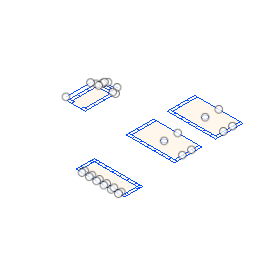
Plano_caja v3 (Autodesk Fusion 360 design; units mm, degrees)
Autodesk Fusion 360 part; units mm, degrees
sketch "Cara_base" plane through (0, 0, 0) normal (0, 1, 0) x (1, 0, 0)
  line L0 (25, -25) -> (78, -25)
  line L1 (78, -25) -> (78, -45)
  line L2 (78, -45) -> (25, -45)
  line L3 (25, -45) -> (25, -25)
  line L4 (25, -45) -> (28, -45)
  line L5 (28, -25) -> (28, -45)
  line L6 (78, -45) -> (75, -45)
  line L7 (75, -25) -> (75, -45)
  line L8 (25, -25) -> (25, -28)
  line L9 (78, -28) -> (25, -28)
  line L10 (25, -45) -> (25, -42)
  line L11 (25, -42) -> (78, -42)
  line L12 (25, -25) -> (25, -30)
  line L13 (25, -30) -> (28, -30)
  line L14 (28, -40) -> (25, -40)
  line L15 (75, -30) -> (78, -30)
  line L16 (75, -40) -> (78, -40)
  line L17 (28, -25) -> (31.5, -25)
  line L18 (31.5, -25) -> (31.5, -28)
  line L19 (75, -28) -> (71.5, -28)
  line L20 (31.5, -28) -> (39.5, -28)
  line L21 (39.4691, -25) -> (39.5, -28)
  line L22 (39.5, -28) -> (47.5, -28)
  line L23 (47.5, -25) -> (47.5, -28)
  line L24 (47.5, -28) -> (55.5, -28)
  line L25 (55.5, -25) -> (55.5, -28)
  line L26 (55.5, -28) -> (63.5, -28)
  line L27 (63.5, -28) -> (63.5, -25)
  line L28 (63.5, -28) -> (71.5, -28)
  line L29 (71.5, -25) -> (71.5, -28)
  line L30 (31.5, -42) -> (31.5, -45)
  line L31 (39.4691, -42) -> (39.5, -45)
  line L32 (47.5, -42) -> (47.5, -45)
  line L33 (55.5, -42) -> (55.5, -45)
  line L34 (63.5, -45) -> (63.5, -42)
  line L35 (71.5, -42) -> (71.5, -45)
  dimension "d1" = 53
  dimension "d2" = 20
  dimension "d3" = 3.5
  dimension "d4" = 3.5
  dimension "d5" = 8
  dimension "d6" = 8
  dimension "d7" = 8
  dimension "d8" = 8
  dimension "d11" = 0
  dimension "d12" = -17
  constraint horizontal L0
  constraint vertical L1
  constraint horizontal L2
  constraint vertical L3
  constraint coincident L2 L4.end
  constraint coincident L0 L5.start
  constraint perpendicular L0 L5
  constraint coincident L2 L6.end
  constraint coincident L0 L7.start
  constraint perpendicular L2 L7
  constraint coincident L3 L8.end
  constraint coincident L1 L9.start
  constraint perpendicular L3 L9
  constraint coincident L3 L10.end
  constraint coincident L1 L11.end
  constraint perpendicular L1 L11
  constraint coincident L3 L12.end
  constraint coincident L5 L13.end
  constraint perpendicular L5 L13
  constraint coincident L3 L14.end
  constraint coincident L5 L14.start
  constraint perpendicular L3 L14
  constraint coincident L7 L15.start
  constraint coincident L1 L15.end
  constraint perpendicular L1 L15
  constraint coincident L7 L16.start
  constraint coincident L1 L16.end
  constraint perpendicular L1 L16
  constraint coincident L0 L17.end
  constraint coincident L9 L18.end
  constraint perpendicular L9 L18
  constraint coincident L7 L19.start
  constraint coincident L9 L19.start
  constraint perpendicular L7 L19
  constraint coincident L9 L20.end
  constraint coincident L0 L21.start
  constraint coincident L9 L22.end
  constraint coincident L0 L23.start
  constraint perpendicular L0 L23
  constraint coincident L9 L24.end
  constraint coincident L0 L25.start
  constraint perpendicular L0 L25
  constraint coincident L9 L26.end
  constraint coincident L0 L27.end
  constraint perpendicular L0 L27
  constraint coincident L0 L29.start
  constraint perpendicular L19 L29
  measures "d1" distance of L0.start L0.end
  measures "d2" distance of L0.start L2.end
  measures "d3" distance of L5.start L17.end
  measures "d4" distance of L19.start L19.end
  measures "d5" distance of L18.end L20.end L0.end
  measures "d6" distance of L20.end L22.end L0.end
  measures "d7" distance of L22.end L24.end L0.end
  measures "d8" distance of L24.end L26.end L0.end
extrude "Extrude1" add sketch "Cara_base" along normal blind 3 contours L0 L3 L5 L8 L9 L12 | L0 L5 L9 L17 L18 | L3 L5 L9 L12 L13 | L5 L7 L9 L11 L19 L20 L22 L24 L26 L28 | L0 L9 L21 L22 L23 | L3 L5 L11 L14 | L2 L3 L4 L5 L10 L11 | L0 L9 L25 L26 L27 | L2 L5 L11 L30 | L0 L7 L9 L19 L29 | L2 L11 L31 L32 | L0 L1 L7 L9 | L1 L7 L9 L15 | L2 L11 L33 L34 | L1 L7 L11 L16 | L2 L7 L11 L35 | L1 L2 L6 L7 L11 makes body 1
sketch "Cara_frontal" plane through (0, 0, 0) normal (0, 1, 0) x (1, 0, 0)
  line L0 (20, 15) -> (73, 15)
  line L1 (73, 15) -> (73, 45)
  line L2 (73, 45) -> (20, 45)
  line L3 (20, 45) -> (20, 15)
  line L4 (20, 15) -> (20, 18)
  line L5 (20, 18) -> (73, 18)
  line L6 (20, 18) -> (26.5, 18)
  line L7 (26.5, 18) -> (26.5, 15)
  line L8 (26.5, 15) -> (34.5, 15)
  line L9 (34.5, 15) -> (34.5, 18)
  line L10 (34.5, 15) -> (42.5, 15)
  line L11 (42.5, 15) -> (50.5, 15)
  line L12 (50.5, 15) -> (58.5, 15)
  line L13 (58.5, 15) -> (66.5, 15)
  line L14 (66.5, 15) -> (73, 15)
  line L15 (42.5, 18) -> (42.5, 15)
  line L16 (50.5, 18) -> (50.5, 15)
  line L17 (58.5, 18) -> (58.5, 15)
  line L18 (66.5, 18) -> (66.5, 15)
  line L19 (20, 45) -> (23, 45)
  line L20 (23, 45) -> (23, 36.5)
  line L21 (23, 36.5) -> (20, 36.5)
  line L22 (23, 36.5) -> (23, 26.5)
  line L23 (23, 26.5) -> (20, 26.5)
  line L24 (23, 26.5) -> (23, 18)
  line L25 (73, 26.5) -> (70, 26.5)
  line L26 (73, 36.5) -> (70, 36.5)
  line L27 (70, 45) -> (70, 18)
  line L28 (23, 45) -> (46.5, 45)
  circle A0 centre (46.5, 30) radius 2.5
  line L29 (26.5, 63) -> (26.5, 60)
  line L30 (73, 90) -> (20, 90)
  circle A1 centre (46.5, 75) radius 2.5
  line L31 (20, 90) -> (23, 90)
  line L32 (73, 60) -> (73, 90)
  line L33 (73, 71.5) -> (70, 71.5)
  line L34 (20, 63) -> (26.5, 63)
  line L35 (23, 81.5) -> (20, 81.5)
  line L36 (66.5, 60) -> (73, 60)
  line L37 (58.5, 60) -> (66.5, 60)
  line L38 (50.5, 60) -> (58.5, 60)
  line L39 (20, 60) -> (73, 60)
  line L40 (23, 81.5) -> (23, 71.5)
  line L41 (42.5, 60) -> (50.5, 60)
  line L42 (50.5, 63) -> (50.5, 60)
  line L43 (73, 81.5) -> (70, 81.5)
  line L44 (23, 71.5) -> (20, 71.5)
  line L45 (70, 90) -> (70, 63)
  line L46 (42.5, 63) -> (42.5, 60)
  line L47 (26.5, 60) -> (34.5, 60)
  line L48 (34.5, 60) -> (42.5, 60)
  line L49 (23, 71.5) -> (23, 63)
  line L50 (34.5, 60) -> (34.5, 63)
  line L51 (20, 60) -> (20, 63)
  line L52 (58.5, 63) -> (58.5, 60)
  line L53 (20, 90) -> (20, 60)
  line L54 (66.5, 63) -> (66.5, 60)
  line L55 (23, 90) -> (46.5, 90)
  line L56 (20, 63) -> (73, 63)
  line L57 (23, 90) -> (23, 81.5)
  dimension "d15" = 30
  dimension "d16" = 53
  dimension "d48" = 5
  dimension "d49" = 30
  dimension "d50" = 53
  dimension "d51" = 5
  constraint horizontal L0
  constraint vertical L1
  constraint horizontal L2
  constraint vertical L3
  constraint coincident L3 L4.end
  constraint coincident L1 L5.end
  constraint perpendicular L1 L5
  constraint coincident L5 L6.end
  constraint coincident L0 L7.end
  constraint perpendicular L0 L7
  constraint coincident L0 L8.end
  constraint coincident L5 L9.end
  constraint perpendicular L5 L9
  constraint coincident L0 L10.end
  constraint coincident L0 L11.end
  constraint coincident L0 L12.end
  constraint coincident L0 L13.end
  constraint coincident L5 L15.start
  constraint coincident L5 L16.start
  constraint coincident L5 L17.start
  constraint coincident L5 L18.start
  constraint coincident L2 L19.end
  constraint perpendicular L2 L20
  constraint coincident L3 L21.end
  constraint perpendicular L3 L21
  constraint perpendicular L21 L22
  constraint coincident L3 L23.end
  constraint perpendicular L3 L23
  constraint coincident L5 L24.end
  constraint coincident L1 L25.start
  constraint perpendicular L1 L25
  constraint coincident L1 L26.start
  constraint perpendicular L1 L26
  constraint coincident L2 L27.start
  constraint coincident L5 L27.end
  constraint perpendicular L5 L27
  constraint perpendicular L27 L28
  constraint horizontal L39
  constraint vertical L32
  constraint horizontal L30
  constraint vertical L53
  constraint coincident L34.start L53
  constraint coincident L56.end L32
  constraint perpendicular L32 L56
  constraint coincident L29.start L56
  constraint coincident L29.end L39
  constraint perpendicular L29 L39
  constraint coincident L47.end L39
  constraint coincident L50.end L56
  constraint perpendicular L50 L56
  constraint coincident L41.start L39
  constraint coincident L38.start L39
  constraint coincident L37.start L39
  constraint coincident L36.start L39
  constraint coincident L46.start L56
  constraint coincident L42.start L56
  constraint coincident L52.start L56
  constraint coincident L54.start L56
  constraint coincident L31.end L30
  constraint perpendicular L30 L57
  constraint coincident L35.end L53
  constraint perpendicular L35 L53
  constraint perpendicular L35 L40
  constraint coincident L44.end L53
  constraint perpendicular L44 L53
  constraint coincident L49.end L56
  constraint coincident L33.start L32
  constraint perpendicular L32 L33
  constraint coincident L43.start L32
  constraint perpendicular L32 L43
  constraint coincident L45.start L30
  constraint coincident L45.end L56
  constraint perpendicular L45 L56
  constraint perpendicular L45 L55
  measures "d15" distance of L0.start L2.end
  measures "d16" distance of L0.start L0.end
  measures "d48" diameter of A0
  measures "d49" distance of L39.start L30.end
  measures "d50" distance of L39.start L32.start
  measures "d51" diameter of A1
extrude "Extrude3" add sketch "Cara_frontal" along normal blind 3 separate body contours L0 L5 L7 L8 L9 | L2 L5 L6 L20 L22 L24 L27 L28 | L3 L21 L22 L23 | L0 L5 L11 L15 L16 | L0 L5 L13 L17 L18 | L1 L25 L26 L27 | A0 makes body 2
sketch "Cara_lateral" plane through (0, 0, 0) normal (0, 1, 0) x (1, 0, 0)
  line L0 (-25, 15) -> (-45, 15)
  line L1 (-45, 15) -> (-45, 45)
  line L2 (-45, 45) -> (-25, 45)
  line L3 (-25, 45) -> (-25, 15)
  line L4 (-45, 15) -> (-40, 15)
  line L5 (-40, 15) -> (-40, 18)
  line L6 (-40, 18) -> (-45, 18)
  line L7 (-25, 18) -> (-30, 18)
  line L8 (-30, 18) -> (-30, 15)
  line L9 (-40, 45) -> (-40, 55)
  line L10 (-30, 55) -> (-30, 45)
  line L11 (-40, 45) -> (-40, 48)
  line L12 (-40, 48) -> (-30, 48)
  line L13 (-37.5, 48.1) -> (-32.5, 48.1)
  line L14 (-32.5, 48.1) -> (-32.5, 51.1)
  line L15 (-32.5, 51.1) -> (-37.5, 51.1)
  line L16 (-37.5, 51.1) -> (-37.5, 48.1)
  line L17 (-42.0655, 51.1) -> (-42.0655, 53.1)
  line L18 (-40, 53.1) -> (-30, 53.1)
  line L19 (-45, 46.8941) -> (-42, 46.8941)
  line L20 (-25, 48.2189) -> (-28, 48.2189)
  line L21 (-42, 45) -> (-42, 18)
  line L22 (-28, 45) -> (-28, 18)
  line L23 (-49.1237, 45) -> (-49.1237, 36.5)
  line L24 (-49.1237, 36.5) -> (-49.1237, 26.5)
  line L25 (-49.1237, 26.5) -> (-49.1237, 18)
  line L26 (-45, 36.5) -> (-42, 36.5)
  line L27 (-45, 26.5) -> (-42, 26.5)
  line L28 (-28, 26.5) -> (-25, 26.5)
  line L29 (-28, 36.5) -> (-25, 36.5)
  dimension "d25" = 20
  dimension "d26" = 30
  dimension "d31" = 2.5
  dimension "d32" = 2.5
  dimension "d35" = 2
  dimension "d38" = 8.5
  dimension "d39" = 10
  dimension "d40" = 8.5
  constraint horizontal L0
  constraint vertical L1
  constraint horizontal L2
  constraint vertical L3
  constraint coincident L0 L4.end
  constraint perpendicular L4 L5
  constraint coincident L1 L6.end
  constraint perpendicular L1 L6
  constraint coincident L3 L7.start
  constraint perpendicular L3 L7
  constraint coincident L0 L8.end
  constraint perpendicular L0 L8
  constraint coincident L2 L9.start
  constraint perpendicular L2 L9
  constraint coincident L2 L10.end
  constraint perpendicular L2 L10
  constraint coincident L9 L11.end
  constraint coincident L10 L12.end
  constraint perpendicular L10 L12
  constraint horizontal L13
  constraint vertical L14
  constraint horizontal L15
  constraint vertical L16
  constraint perpendicular L15 L17
  constraint coincident L9 L18.start
  constraint coincident L10 L18.end
  constraint perpendicular L10 L18
  constraint perpendicular L10 L19
  constraint perpendicular L3 L20
  constraint coincident L2 L21.start
  constraint coincident L6 L21.end
  constraint perpendicular L6 L21
  constraint coincident L2 L22.start
  constraint coincident L7 L22.end
  constraint perpendicular L7 L22
  constraint perpendicular L2 L23
  constraint perpendicular L2 L24
  constraint perpendicular L2 L25
  constraint coincident L1 L26.start
  constraint coincident L21 L26.end
  constraint perpendicular L21 L26
  constraint coincident L1 L27.start
  constraint coincident L21 L27.end
  constraint perpendicular L21 L27
  constraint coincident L22 L28.start
  constraint coincident L3 L28.end
  constraint perpendicular L3 L28
  constraint coincident L22 L29.start
  constraint coincident L3 L29.end
  constraint perpendicular L3 L29
  measures "d25" distance of L0.start L0.end
  measures "d26" distance of L0.start L2.end
  measures "d31" distance of L9 L16
  measures "d32" distance of L10 L14
  measures "d35" distance of L17.start L17.end
  measures "d38" distance of L23.start L23.end
  measures "d39" distance of L23.end L24.end
  measures "d40" distance of L24.end L25.end
extrude "Extrude2" add sketch "Cara_lateral" along normal blind 3 separate body contours L0 L2 L5 L6 L7 L8 L21 L22 | L3 L7 L22 L28 | L2 L3 L22 L29 | L1 L6 L21 L27 | L1 L2 L21 L26 | L2 L9 L10 L11 L12 | L9 L10 L12 L18 makes body 3
extrude "Extrude4" add sketch "Cara_frontal" along normal blind 3 separate body contours L29 L39 L47 L50 L56 | L30 L34 L40 L45 L49 L55 L56 L57 | L35 L40 L44 L53 | L39 L41 L42 L46 L56 | L37 L39 L52 L54 L56 | L32 L33 L43 L45 makes body 4
copy_body "Body->Comp1" bodies 1 removing the originals makes body 5 in component "Cara_Base"
copy_body "Body->Comp2" bodies 2 removing the originals makes body 6 in component "Frontal_tapa"
copy_body "Body->Comp3" bodies 4 removing the originals makes body 7 in component "Frontal_frente"
copy_body "Body->Comp4" bodies 3 removing the originals makes body 8 in component "Lateral"
sketch "Sketch4" plane through (0, 0, 0) normal (0, 1, 0) x (1, 0, 0)
  line L0 (-25, -15) -> (-30, -15)
  line L1 (-30, -15) -> (-30, -28)
  line L2 (-30, -28) -> (-25, -28)
  line L3 (-25, -28) -> (-25, -15)
  dimension "d56" = 5
  dimension "d57" = 13
  constraint horizontal L0
  constraint vertical L1
  constraint horizontal L2
  constraint vertical L3
  measures "d56" distance of L0.start L0.end
  measures "d57" distance of L0.start L2.end
extrude "Extrude5" add sketch "Sketch4" along normal blind 3 separate body makes body 9
copy_body "Body->Comp5" bodies 9 removing the originals makes body 10 in component "Pasador"
component "Cara_Base" placed x (1, 0, 0) y (0, 1, 0) z (0, 0, 1) at (0, 0, 0)
component "Frontal_tapa" placed x (1, 0, 0) y (0, 1, 0) z (0, 0, 1) at (0, 0, 0)
component "Frontal_frente" placed x (1, 0, 0) y (0, 1, 0) z (0, 0, 1) at (0, 0, 0)
component "Lateral" placed x (1, 0, 0) y (0, 1, 0) z (0, 0, 1) at (0, 0, 0)
component "Pasador" placed x (1, 0, 0) y (0, 1, 0) z (0, 0, 1) at (0, 0, 0)
equation "d38 = ( 17 / 2 ) * 1 mm"
equation "d57 = 3 mm + 10 mm"
named bodies: "Cara_Base", "Lateral", "Frontal_tapa", "Frontal_frente", "Pasador"
